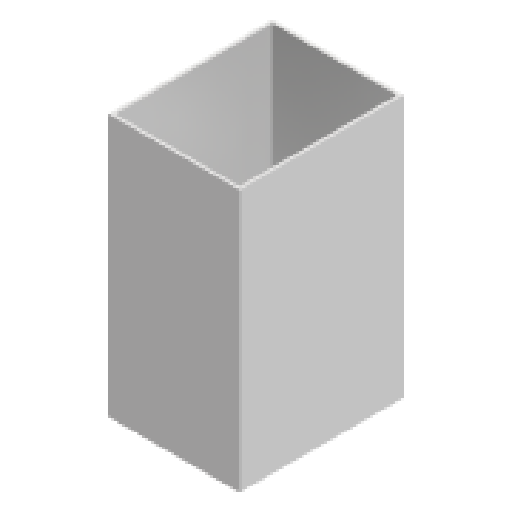
# Autodesk Inventor part: Reflector
Saved by Autodesk Inventor 2026.1 (Build 301233000, 233)
## iProperties
Created: 2026-03-01
Part Number: Reflector
Material: Generic
Document SubType Name: Modeling
Designer: aleja
Density: 1 g/cm^3
Appearance: Default
Author: aleja
Autodesk Inventor part; units mm, degrees
ref_plane "YZ Plane" through (0, 0, 0) normal (1, 0, 0) x (0, 1, 0)
ref_plane "XZ Plane" through (0, 0, 0) normal (0, 1, 0) x (-1, 0, 0)
ref_plane "XY Plane" through (0, 0, 0) normal (0, 0, 1) x (1, 0, 0)
sketch "Sketch1" plane through (0, 0, 0) normal (0, 0, 1) x (1, 0, 0)
  line L0 (-60, 75) -> (60, 75)
  line L1 (60, 75) -> (60, -75)
  line L2 (60, -75) -> (-60, -75)
  line L3 (-60, -75) -> (-60, 75)
  line L4 (-60, 75) -> (60, -75) construction
  line L5 (60, 75) -> (-60, -75) construction
  line L6 (60, 75) -> (60, -75) projected
  line L7 (40, -75) -> (-60, -75) projected
  line L8 (57, -72) -> (57, 72)
  line L9 (57, 72) -> (-57, 72)
  line L10 (-57, 72) -> (-57, -72)
  line L11 (-57, -72) -> (57, -72)
  point P0 (0, 0)
  dimension "d0" = 3
  constraints: 20 end point, 4 parallel, 2 collinear, 2 midpoint, 2 perpendicular, 1 horizontal, 3 other
  measures "d0" distance between parallel lines of L1 L8
extrude "Extrusion1" add sketch "Sketch1" along normal blind 240
body "Solid1"
